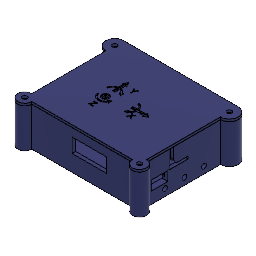
Main_Board_Box v1 (Autodesk Fusion 360 design; units mm, degrees)
part number: Utils
Autodesk Fusion 360 part; units mm, degrees
sketch "Sketch1" plane through (0, 0, 0) normal (0, 1, 0) x (1, 0, 0) in component "Bottom"
  line L0 (43.255, -32.62) -> (-43.255, -32.62) construction
  line L1 (-43.255, -32.62) -> (-43.255, 32.62) construction
  line L2 (-43.255, 32.62) -> (43.255, 32.62) construction
  line L3 (43.255, 32.62) -> (43.255, -32.62) construction
  line L4 (43.255, -32.62) -> (-43.255, 32.62) construction
  line L5 (-43.255, -32.62) -> (43.255, 32.62) construction
  line L6 (43.5, -33) -> (-43.5, -33)
  line L7 (-43.5, -33) -> (-43.5, 33)
  line L8 (-43.5, 33) -> (43.5, 33)
  line L9 (43.5, 33) -> (43.5, -33)
  line L10 (43.5, -33) -> (-43.5, 33) construction
  line L11 (-43.5, -33) -> (43.5, 33) construction
  line L12 (-43.255, -32.62) -> (-29.285, -32.62)
  line L13 (-29.285, -32.62) -> (-29.285, -28.81) construction
  circle A0 centre (-29.285, -28.81) radius 1.1
  line L14 (-29.285, -28.81) -> (29.135, -28.81) construction
  circle A1 centre (29.135, -28.81) radius 1.1
  line L15 (-29.285, -28.81) -> (-29.285, 28.34) construction
  line L16 (-43.255, 28.34) -> (-25.475, 28.34) construction
  circle A2 centre (-25.475, 28.34) radius 1.1
  line L17 (-25.475, 28.34) -> (15.165, 28.34) construction
  circle A3 centre (15.165, 28.34) radius 1.1
  line L18 (-43.255, 32.62) -> (-41.255, 32.62) construction
  line L19 (-41.255, 32.62) -> (-41.255, 40.62) construction
  line L20 (-41.255, 40.62) -> (-10.255, 40.62) construction
  line L21 (-10.255, 40.62) -> (-10.255, 32.62) construction
  line L22 (34.135, -33) -> (24.135, -33)
  line L23 (24.135, -33) -> (24.135, -27.62)
  line L24 (27.135, -24.62) -> (31.135, -24.62)
  line L25 (34.135, -27.62) -> (34.135, -33)
  arc A4 (27.135, -24.62) -> (24.135, -27.62) centre (27.135, -27.62) ccw
  arc A5 (34.135, -27.62) -> (31.135, -24.62) centre (31.135, -27.62) ccw
  line L26 (-24.285, -33) -> (-34.285, -33)
  line L27 (-34.285, -33) -> (-34.285, -27.62)
  line L28 (-31.285, -24.62) -> (-27.285, -24.62)
  line L29 (-24.285, -27.62) -> (-24.285, -33)
  arc A6 (-24.285, -27.62) -> (-27.285, -24.62) centre (-27.285, -27.62) ccw
  arc A7 (-31.285, -24.62) -> (-34.285, -27.62) centre (-31.285, -27.62) ccw
  line L30 (-15.475, 33) -> (-35.475, 33)
  line L31 (-35.475, 33) -> (-35.475, 26.68)
  line L32 (-32.475, 23.68) -> (-18.475, 23.68)
  line L33 (-15.475, 26.68) -> (-15.475, 33)
  arc A8 (-18.475, 23.68) -> (-15.475, 26.68) centre (-18.475, 26.68) ccw
  arc A9 (-35.475, 26.68) -> (-32.475, 23.68) centre (-32.475, 26.68) ccw
  line L34 (25.165, 33) -> (5.165, 33)
  line L35 (5.165, 33) -> (5.165, 26.68)
  line L36 (8.165, 23.68) -> (22.165, 23.68)
  line L37 (25.165, 26.68) -> (25.165, 33)
  arc A10 (22.165, 23.68) -> (25.165, 26.68) centre (22.165, 26.68) ccw
  arc A11 (5.165, 26.68) -> (8.165, 23.68) centre (8.165, 26.68) ccw
  line L38 (45.5, -35) -> (-45.5, -35)
  line L39 (-45.5, -35) -> (-45.5, 35)
  line L40 (45.5, 35) -> (45.5, -35)
  line L41 (45.5, -35) -> (-45.5, 35) construction
  line L42 (-45.5, -35) -> (45.5, 35) construction
  line L43 (-43.255, 35) -> (-43.255, 42.5)
  line L44 (-43.255, 42.5) -> (-8.255, 42.5)
  line L45 (-45.5, 35) -> (-43.255, 35)
  line L46 (-8.255, 35) -> (45.5, 35) construction
  line L47 (48.5, 38) -> (-48.5, -38) construction
  line L48 (-48.5, 38) -> (48.5, -38) construction
  line L49 (-5.255, 45.5) -> (-46.255, 45.5)
  circle A12 centre (48.5, 38) radius 1.4
  circle A13 centre (-48.5, 38) radius 1.4
  circle A14 centre (48.5, -38) radius 1.4
  circle A15 centre (-48.5, -38) radius 1.4
  arc A16 (42.5, -38) -> (48.5, -32) centre (48.5, -38) ccw
  line L50 (48.5, -32) -> (48.5, 30.5)
  arc A17 (-48.5, -32) -> (-42.5, -38) centre (-48.5, -38) ccw
  line L51 (-46.255, 45.5) -> (-48.5, 45.5)
  arc A18 (-48.5, 45.5) -> (-48.5, 30.5) centre (-48.5, 38) ccw
  line L52 (-42.5, -38) -> (42.5, -38)
  line L53 (-48.5, 30.5) -> (-48.5, -32)
  line L54 (-5.255, 45.5) -> (48.5, 45.5)
  line L55 (-8.255, 42.5) -> (45.5, 42.5)
  arc A19 (48.5, 30.5) -> (48.5, 45.5) centre (48.5, 38) ccw
  arc A20 (45.5, 41) -> (45.5, 35) centre (48.5, 38) ccw
  line L56 (45.5, 42.5) -> (45.5, 41)
  point P0 (29.135, -28.81)
  point P1 (-29.285, -28.81)
  point P2 (-25.475, 28.34)
  point P3 (15.165, 28.34)
  dimension "d1" = 86.51
  dimension "d2" = 65.24
  dimension "d3" = 87
  dimension "d4" = 66
  dimension "d5" = 13.97
  dimension "d6" = 3.81
  dimension "d7" = 2.2
  dimension "d8" = 58.42
  dimension "d9" = 2.2
  dimension "d10" = 57.15
  dimension "d11" = 17.78
  dimension "d12" = 2.2
  dimension "d13" = 40.64
  dimension "d14" = 2.2
  dimension "d15" = 2
  dimension "d16" = 8
  dimension "d17" = 31
  dimension "d19" = 3
  dimension "d20" = 3
  dimension "d22" = 3
  dimension "d23" = 3
  dimension "d25" = 3
  dimension "d26" = 3
  dimension "d28" = 3
  dimension "d29" = 3
  dimension "d30" = 91
  dimension "d31" = 70
  dimension "d33" = 7.5
  dimension "d34" = 97
  dimension "d35" = 76
  dimension "d39" = 2.8
  dimension "d40" = 2.8
  dimension "d41" = 2.8
  dimension "d42" = 2.8
  dimension "d43" = 6
  dimension "d44" = 6
  constraint perpendicular L0 L1
  constraint parallel L0 L2
  constraint parallel L1 L3
  constraint horizontal L0
  constraint coincident L4 origin
  constraint coincident L5 origin
  constraint perpendicular L6 L7
  constraint parallel L6 L8
  constraint parallel L7 L9
  constraint horizontal L6
  constraint coincident L10 origin
  constraint coincident L11 origin
  constraint perpendicular L1 L12
  constraint vertical L13
  constraint coincident P1 L13.end
  constraint horizontal L14
  constraint coincident P0 L14.end
  constraint vertical L15
  constraint coincident L1 L16.start
  constraint perpendicular L1 L16
  constraint coincident P2 L16.end
  constraint horizontal L17
  constraint coincident P3 L17.end
  constraint perpendicular L1 L18
  constraint perpendicular L2 L19
  constraint perpendicular L19 L20
  constraint coincident L2 L21.end
  constraint perpendicular L2 L21
  constraint perpendicular L22 L23
  constraint parallel L22 L24
  constraint parallel L23 L25
  constraint horizontal L22
  constraint coincident L6 L22.start
  constraint tangent L23 A4
  constraint tangent L24 A4
  constraint tangent L25 A5
  constraint tangent L24 A5
  constraint perpendicular L26 L27
  constraint parallel L26 L28
  constraint parallel L27 L29
  constraint horizontal L26
  constraint coincident L6 L26.start
  constraint tangent L29 A6
  constraint tangent L28 A6
  constraint tangent L27 A7
  constraint tangent L28 A7
  constraint perpendicular L30 L31
  constraint parallel L30 L32
  constraint parallel L31 L33
  constraint horizontal L30
  constraint coincident L8 L30.start
  constraint tangent L32 A8
  constraint tangent L33 A8
  constraint tangent L32 A9
  constraint tangent L31 A9
  constraint perpendicular L34 L35
  constraint parallel L34 L36
  constraint parallel L35 L37
  constraint horizontal L34
  constraint coincident L8 L34.start
  constraint tangent L36 A10
  constraint tangent L37 A10
  constraint tangent L36 A11
  constraint tangent L35 A11
  constraint perpendicular L38 L39
  constraint parallel L38 L45
  constraint parallel L39 L40
  constraint horizontal L38
  constraint coincident L41 origin
  constraint coincident L42 origin
  constraint perpendicular L20 L43
  constraint perpendicular L43 L44
  constraint collinear L45 L46
  constraint coincident L47 origin
  constraint coincident L48 origin
  constraint coincident L47.start A12.centre
  constraint coincident L48.start A13.centre
  constraint coincident L48.end A14.centre
  constraint coincident L47.end A15.centre
  constraint perpendicular L40 L54
  constraint perpendicular L40 L55
  constraint perpendicular L55 L56
  measures "d1" distance of L1.end L2.end
  measures "d2" distance of L0.end L1.end
  measures "d3" distance of L7.end L8.end
  measures "d4" distance of L6.end L7.end
  measures "d5" distance of L0.end L12.end
  measures "d6" distance of L12.end P1
  measures "d7" diameter of A0
  measures "d8" distance of P1 P0
  measures "d9" diameter of A1
  measures "d10" distance of P1 L15.end
  measures "d11" distance of L16.start P2
  measures "d12" diameter of A2
  measures "d13" distance of P2 P3
  measures "d14" diameter of A3
  measures "d15" distance of L1.end L18.end
  measures "d16" distance of L18.end L19.end
  measures "d17" distance of L19.end L20.end
  measures "d19" radius of A4
  measures "d20" radius of A5
  measures "d22" radius of A6
  measures "d23" radius of A7
  measures "d25" radius of A8
  measures "d26" radius of A9
  measures "d28" radius of A10
  measures "d29" radius of A11
  measures "d30" distance of L39.end L40.start
  measures "d31" distance of L38.end L39.end
  measures "d33" distance of L43.start L43.end
  measures "d34" distance of L47.end L48.end
  measures "d35" distance of L48.start L47.end
  measures "d39" diameter of A12
  measures "d40" diameter of A13
  measures "d41" diameter of A14
  measures "d42" diameter of A15
  measures "d43" radius of A16
  measures "d44" radius of A17
extrude "Extrude1" add sketch "Sketch1" against normal blind 2 from surface at -8 contours L6 L7 L8 L9 L23 L24 L25 A4 A5 L27 L28 L29 A6 A7 L31 L32 L33 A8 A9 L35 L36 L37 A10 A11 | L6 L22 L23 L24 L25 A4 A5 | L8 L34 L35 L36 L37 A10 A11 | L6 L26 L27 L28 L29 A6 A7 | L8 L30 L31 L32 L33 A8 A9 | L38 L39 L40 L43 L44 L45 L55 A20 L56 | L49 A16 L50 A17 L51 A18 L52 L53 L54 A19 makes body 1 in component "Bottom"
extrude "Extrude2" add sketch "Sketch1" against normal blind 8 contours L6 L22 L23 L24 L25 A4 A5 | L8 L34 L35 L36 L37 A10 A11 | L6 L26 L27 L28 L29 A6 A7 | L8 L30 L31 L32 L33 A8 A9 | L38 L39 L40 L43 L44 L45 L55 A20 L56 | L49 A16 L50 A17 L51 A18 L52 L53 L54 A19 bodies 1 in component "Bottom"
extrude "Extrude3" add sketch "Sketch1" along normal blind 2 contours L38 L39 L40 L43 L44 L45 L55 A20 L56 bodies 1 in component "Bottom"
extrude "Extrude4" add sketch "Sketch1" along normal blind 23 contours L49 A16 L50 A17 L51 A18 L52 L53 L54 A19 bodies 1 in component "Bottom"
sketch "Sketch1 (2)" plane through (0, 23, 0) normal (0, 1, 0) x (-1, 0, 0) in component "Top"
  circle A0 centre (-48.5, 38) radius 1.4 construction
  circle A1 centre (48.5, 38) radius 1.4 construction
  circle A2 centre (-48.5, -38) radius 1.4 construction
  line L0 (43.255, -42.5) -> (-45.5, -42.5)
  line L1 (-45.5, -42.5) -> (-45.5, -41)
  arc A3 (-45.5, -41) -> (-45.5, -35) centre (-48.5, -38) ccw
  line L2 (-45.5, -35) -> (-45.5, 35)
  line L3 (-45.5, 35) -> (45.5, 35)
  line L4 (45.5, 35) -> (45.5, -35)
  line L5 (45.5, -35) -> (43.255, -35)
  line L6 (43.255, -35) -> (43.255, -42.5)
  circle A4 centre (48.5, -38) radius 1.4 construction
  line L7 (-48.5, -45.5) -> (48.5, -45.5)
  arc A5 (48.5, -45.5) -> (48.5, -30.5) centre (48.5, -38) ccw
  line L8 (48.5, -30.5) -> (48.5, 32)
  arc A6 (48.5, 32) -> (42.5, 38) centre (48.5, 38) ccw
  line L9 (42.5, 38) -> (-42.5, 38)
  arc A7 (-42.5, 38) -> (-48.5, 32) centre (-48.5, 38) ccw
  line L10 (-48.5, 32) -> (-48.5, -30.5)
  arc A8 (-48.5, -30.5) -> (-48.5, -45.5) centre (-48.5, -38) ccw
  line L11 (45.5, 35) -> (45, 35)
  line L12 (45.5, 34.5) -> (45.5, 35)
  line L13 (-45.5, 35) -> (-45, 35)
  line L14 (-45.5, 34.5) -> (-45.5, 35)
  line L15 (45.5, -35) -> (45, -35)
  line L16 (45.5, -34.5) -> (45.5, -35)
  line L17 (42.755, -35) -> (42.755, -34.5)
  line L18 (42.755, -34.5) -> (43.255, -34.5)
  line L19 (43.255, -42.5) -> (42.755, -42.5)
  line L20 (43.255, -42) -> (43.255, -42.5)
  line L21 (-45.5, -34.5) -> (-45.5, -35)
  line L22 (-45, -41.5) -> (-45, -42)
  line L23 (-45, -42.5) -> (-45.5, -42.5)
  line L24 (-45.5, -42.5) -> (-45.5, -41)
  arc A9 (-45, -41.5) -> (-45, -34.5) centre (-48.5, -38) ccw
  line L25 (-45, -42) -> (42.755, -42)
  line L26 (42.755, -42) -> (42.755, -35)
  line L27 (43.255, -34.5) -> (45, -34.5)
  line L28 (45, -34.5) -> (45, 34.5)
  line L29 (45, 34.5) -> (-45, 34.5)
  line L30 (-45, 34.5) -> (-45, -34.5)
  line L31 (-47, -42.5) -> (-47, -40)
  line L32 (40.755, -40) -> (40.755, -35)
  line L33 (40.755, -35) -> (40.755, -32.5)
  line L34 (40.755, -32.5) -> (43, -32.5)
  line L35 (43, -32.5) -> (43, 32.5)
  line L36 (43, 32.5) -> (-43, 32.5)
  line L37 (-43, 32.5) -> (-43, -33.7516)
  arc A10 (-41.8443, -40) -> (-43, -33.7516) centre (-48.5, -38) ccw
  line L38 (-47, -40) -> (-44.7583, -40)
  line L39 (-41.8443, -40) -> (40.755, -40)
  circle A11 centre (48.5, -38) radius 2
  circle A12 centre (48.5, 38) radius 2
  circle A13 centre (-48.5, 38) radius 2
  circle A14 centre (-48.5, -38) radius 2
  dimension "d56" = 0.5
  dimension "d57" = 0.5
  dimension "d58" = 0.5
  dimension "d59" = 0.5
  dimension "d60" = 0.5
  dimension "d61" = 0.5
  dimension "d62" = 0.5
  dimension "d63" = 0.5
  dimension "d64" = 0.5
  dimension "d65" = 0.5
  dimension "d67" = 0.5
  dimension "d70" = 0.5
  dimension "d76" = 4
  dimension "d77" = 4
  dimension "d78" = 4
  dimension "d79" = 4
  constraint horizontal L11
  constraint vertical L12
  constraint coincident L3.end L4.start
  constraint horizontal L13
  constraint vertical L14
  constraint coincident L2.end L3.start
  constraint horizontal L15
  constraint vertical L16
  constraint coincident L4.end L5.start
  constraint vertical L17
  constraint horizontal L18
  constraint horizontal L19
  constraint vertical L20
  constraint coincident L0.start L6.end
  constraint vertical L21
  constraint coincident A3.end L2.start
  constraint vertical L22
  constraint horizontal L23
  constraint vertical L24
  constraint coincident L1.end A3.start
  constraint coincident L0 L23.start
  constraint coincident A2.centre A3.centre
  constraint parallel L25 L38
  constraint parallel L26 L32
  constraint parallel L17 L33
  constraint parallel L18 L34
  constraint parallel L28 L35
  constraint parallel L29 L36
  constraint parallel L30 L37
  constraint coincident A10.start L38
  constraint collinear L38 L39
  constraint coincident A3 L38.end
  constraint concentric A4 A11
  constraint concentric A1 A12
  constraint concentric A0 A13
  constraint concentric A9 A14
  measures "d56" distance of L3.end L12.start
  measures "d57" distance of L3.end L11.end
  measures "d58" distance of L2.end L14.start
  measures "d59" distance of L2.end L13.end
  measures "d60" distance of L4.end L15.end
  measures "d61" distance of L4.end L16.start
  measures "d62" distance of L5.end L17.start
  measures "d63" distance of L5.end L18.end
  measures "d64" distance of L0.start L19.end
  measures "d65" distance of L0.start L20.start
  measures "d67" distance of A3.end L21.start
  measures "d70" distance of L23.start L22.end
  measures "d76" diameter of A11
  measures "d77" diameter of A12
  measures "d78" diameter of A13
  measures "d79" diameter of A14
extrude "Extrude1'" add sketch "Sketch1 (2)" against normal blind 3 separate body contours L17 L18 L22 A9 L25 L26 L27 L28 L29 L30 makes body 2 in component "Top"
extrude "Extrude2'" add sketch "Sketch1 (2)" along normal blind 2 contours L0 L1 A3 L2 L3 L4 L5 L6 L11 L12 L13 L14 L15 L16 L19 L20 L21 L23 L24 | L7 A5 L8 A6 L9 A7 L10 A8 | L17 L18 L22 A9 L25 L26 L27 L28 L29 L30 | L32 L33 L34 L35 L36 L37 A10 L39 bodies 2 in component "Top"
sketch "Sketch2" plane through (48.5, 0, 0) normal (1, 0, 0) x (0, 0, -1) in component "Bottom"
  line L0 (-32, 23) -> (-32, -10)
  line L1 (-32, -10) -> (30.5, -10)
  line L2 (30.5, -10) -> (30.5, 23)
  line L3 (30.5, 23) -> (-32, 23)
  line L4 (-32, 0) -> (30.5, 0)
  line L5 (33, 2) -> (-33, 2) construction
  line L6 (35, 0) -> (-35, 0)
  line L7 (-33, -8) -> (-33, 2)
  line L8 (-33, 0) -> (-28, 0)
  line L9 (-33, 0) -> (-14, 0)
  line L10 (-28, 0) -> (-14, 0)
  line L11 (-14, 0) -> (-14, 8)
  line L12 (-14, 8) -> (-28, 8)
  line L13 (-28, 8) -> (-28, 0)
  line L14 (-13, 8) -> (3, 8)
  line L15 (3, 8) -> (3, 10)
  line L16 (3, 10) -> (-5.4645, 10)
  line L17 (-13, 10) -> (-13, 8)
  line L18 (-13, 8) -> (-9, 8)
  line L19 (-9, 23) -> (-13, 23)
  line L20 (-13, 23) -> (-13, 8)
  arc A0 (-9, 13.5355) -> (-5.4645, 10) centre (-5.4645, 13.5355) ccw
  line L21 (-9, 13.5355) -> (-9, 23)
  line L22 (33, 2) -> (33, -8)
  line L23 (33, -8) -> (-33, -8)
  line L24 (-33, -8) -> (-33, 2)
  line L25 (-33, 2) -> (33, 2)
  line L26 (-33, 0) -> (33, -8) construction
  line L27 (33, 0) -> (-33, -8) construction
  line L28 (0, 0) -> (-33, -8) construction
  line L29 (-33, 0) -> (0, -8) construction
  line L30 (33, 0) -> (0, -8) construction
  line L31 (0, 0) -> (33, -8) construction
  circle A1 centre (-16.5, -4) radius 2
  circle A2 centre (0, -4) radius 2
  circle A3 centre (16.5, -4) radius 2
  dimension "d82" = 5
  dimension "d83" = 19
  dimension "d84" = 8
  dimension "d88" = 1
  dimension "d89" = 16
  dimension "d90" = 2
  dimension "d91" = 4
  dimension "d92" = 4
  dimension "d93" = 4
  dimension "d94" = 4
  dimension "d69_1" = 0
  dimension "d73_1" = 0
  dimension "d129_1" = 0
  constraint coincident L6 L8.start
  constraint coincident L7 L8.start
  constraint perpendicular L7 L8
  constraint parallel L6 L9
  constraint horizontal L10
  constraint vertical L11
  constraint horizontal L12
  constraint vertical L13
  constraint horizontal L14
  constraint vertical L15
  constraint horizontal L16
  constraint vertical L17
  constraint horizontal L18
  constraint horizontal L19
  constraint vertical L20
  constraint coincident L3 L19.start
  constraint tangent L16 A0
  constraint coincident L22.end L23.start
  constraint coincident L6 L27.start
  constraint coincident L22 L27.start
  constraint coincident L7.start L23.end
  constraint coincident L28.start L31.start
  constraint midpoint L23 L29.end
  constraint midpoint L28 A1.centre
  constraint midpoint L26 A2.centre
  constraint midpoint L30 A3.centre
  measures "d82" distance of L8.start L8.end
  measures "d83" distance of L8.start L9.end
  measures "d84" distance of L8.end L12.end
  measures "d88" distance of L11.end L14.start
  measures "d89" distance of L14.start L14.end
  measures "d90" distance of L14.start L17.start
  measures "d91" distance of L14.start L18.end
  measures "d92" diameter of A1
  measures "d93" diameter of A2
  measures "d94" diameter of A3
extrude "Extrude5" cut sketch "Sketch2" against normal blind 10 contours L4 L6 L9 L10 L11 L13 L25 | L11 L12 L13 L25 bodies 1 in component "Bottom"
extrude "Extrude6" cut sketch "Sketch2" against normal blind 5 contours L3 L14 L15 L16 L17 L18 L19 L20 A0 L21 bodies 1 in component "Bottom"
extrude "Extrude7" cut sketch "Sketch2" against normal blind 107 contours A1 | A2 | A3 bodies 1 in component "Bottom"
sketch "Sketch3" plane through (0, 0, 38) normal (0, 0, 1) x (1, 0, 0) in component "Bottom"
  line L0 (-42.5, 23) -> (-42.5, -10)
  line L1 (-42.5, -10) -> (42.5, -10)
  line L2 (42.5, -10) -> (42.5, 23)
  line L3 (42.5, 23) -> (-42.5, 23)
  line L4 (-42.5, 0) -> (42.5, 0)
  line L5 (43.5, 0) -> (20.5, 0)
  line L6 (20.5, 0) -> (20.5, 4)
  line L7 (43.5, 0) -> (-8.5, 0)
  line L8 (20.5, 4) -> (-8.5, 4)
  line L9 (-8.5, 4) -> (-8.5, 16)
  line L10 (-8.5, 16) -> (20.5, 16)
  line L11 (20.5, 16) -> (20.5, 4)
  point P0 (43.5, 0)
  dimension "d99" = 23
  dimension "d100" = 4
  dimension "d101" = 52
  dimension "d102" = 12
  constraint coincident P0 L5.start
  constraint perpendicular L2 L5
  constraint perpendicular L4 L6
  constraint perpendicular L6 L7
  constraint horizontal L8
  constraint vertical L9
  constraint horizontal L10
  constraint vertical L11
  measures "d99" distance of P0 L5.end
  measures "d100" distance of L5.end L6.end
  measures "d101" distance of P0 L7.end
  measures "d102" distance of L6.end L10.end
extrude "Extrude8" cut sketch "Sketch3" against normal blind 7 contours L8 L9 L10 L11 bodies 1 in component "Bottom"
sketch "Sketch6" plane through (0, 25, 0) normal (0, 1, 0) x (-1, 0, 0) in component "Utils"
  line L0 (15.1244, 3.1244) -> (21.0332, 4.1662) construction
  line L1 (15.1244, 3.1244) -> (15.1244, 8.1244) construction
  line L2 (15.1244, 3.1244) -> (10.7942, 5.6244) construction
  line L3 (15.1244, 3.1244) -> (15.1244, 8.1244) construction
  line L4 (15.1244, 3.1244) -> (15.1244, 9.1244) construction
  line L5 (9.0622, 6.6244) -> (9.0622, 3.6244)
  line L6 (15.1244, 3.1244) -> (20.0484, 3.9926) construction
  line L7 (11.6603, 5.1244) -> (9.0622, 3.6244)
  line L8 (15.1244, 6.1244) -> (15.1244, 8.1244)
  arc A0 (15.1244, 8.1244) -> (10.7942, 5.6244) centre (15.1244, 3.1244) ccw
  line L9 (15.1244, 3.1244) -> (15.1244, 6.1244) construction
  line L10 (15.1244, 8.1244) -> (15.1244, 9.1244) construction
  line L11 (20.0484, 3.9926) -> (21.0332, 4.1662)
  line L12 (9.9282, 6.1244) -> (9.0622, 6.6244)
  circle A1 centre (15.1244, 3.1244) radius 1
  arc A2 (21.0332, 4.1662) -> (15.1244, 9.1244) centre (15.1244, 3.1244) ccw
  line L13 (10.7942, 5.6244) -> (11.6603, 5.1244)
  circle A3 centre (15.1244, 3.1244) radius 3
  arc A4 (15.1244, 9.1244) -> (9.9282, 6.1244) centre (15.1244, 3.1244) ccw
  arc A5 (20.0484, 3.9926) -> (15.1244, 8.1244) centre (15.1244, 3.1244) ccw
  line L14 (15.1244, 3.1244) -> (15.1244, 9.1244) construction
  line L15 (15.1244, 3.1244) -> (9.9282, 6.1244) construction
  circle A6 centre (15.1244, 3.1244) radius 2
  line L16 (16.9519, 15.6272) -> (13.5564, 15.6272) construction
  line L17 (13.5564, 15.6272) -> (13.5564, 9.6272) construction
  line L18 (13.5564, 9.6272) -> (16.9519, 9.6272) construction
  line L19 (16.9519, 9.6272) -> (16.9519, 15.6272) construction
  line L20 (0, 0) -> (-4, 0) construction
  line L21 (-4, 0) -> (-4, -1)
  line L22 (-4, 0) -> (-4, 1)
  line L23 (-4, -1) -> (-15, -1)
  line L24 (-15, -1) -> (-15, -2)
  line L25 (-4, 1) -> (-15, 1)
  line L26 (-15, 1) -> (-15, 2)
  line L27 (-15, -2) -> (-18.4641, 0)
  line L28 (-15, 2) -> (-18.4641, 0)
  line L29 (-8.0481, 8.6272) -> (-11.9856, 8.6272) construction
  line L30 (-11.9856, 8.6272) -> (-11.9856, 2.6272) construction
  line L31 (-11.9856, 2.6272) -> (-8.0481, 2.6272) construction
  line L32 (-8.0481, 2.6272) -> (-8.0481, 8.6272) construction
  arc A7 (-5.5622, 4.2679) -> (-7.6024, 2.0322) centre (-3.0622, -0.0622) ccw
  line L33 (-6.5622, 6) -> (-3.5622, 6)
  line L34 (-3.9304, -4.9862) -> (-4.1041, -5.971)
  arc A8 (-6.0622, 5.134) -> (-8.5104, 2.4511) centre (-3.0622, -0.0622) ccw
  line L35 (-6.0622, 5.134) -> (-6.5622, 6)
  line L36 (-5.0622, 3.4019) -> (-3.5622, 6)
  line L37 (-5.5622, 4.2679) -> (-5.0622, 3.4019)
  line L38 (16.3923, -4.1436) -> (16.3923, -13.1436)
  line L39 (17.3923, -13.1436) -> (15.3923, -16.6077)
  line L40 (16.3923, -13.1436) -> (17.3923, -13.1436)
  line L41 (14.3923, -4.1436) -> (14.3923, -13.1436)
  line L42 (14.3923, -13.1436) -> (13.3923, -13.1436)
  arc A9 (10.2583, -6.2058) -> (12.9412, -8.654) centre (15.4545, -3.2058) ccw
  line L43 (20.3785, -4.074) -> (21.3633, -4.2477)
  line L44 (15.3923, -4.1436) -> (14.3923, -4.1436)
  line L45 (11.9904, -5.2058) -> (9.3923, -3.7058)
  arc A10 (11.1244, -5.7058) -> (13.3601, -7.746) centre (15.4545, -3.2058) ccw
  line L46 (13.3923, -13.1436) -> (15.3923, -16.6077)
  line L47 (15.3923, -4.1436) -> (16.3923, -4.1436)
  line L48 (11.1244, -5.7058) -> (11.9904, -5.2058)
  line L49 (9.3923, -6.7058) -> (9.3923, -3.7058)
  line L50 (10.2583, -6.2058) -> (9.3923, -6.7058)
  line L51 (8.9519, -10.3728) -> (5.0144, -10.3728) construction
  line L52 (5.0144, -10.3728) -> (5.0144, -16.3728) construction
  line L53 (5.0144, -16.3728) -> (8.9519, -16.3728) construction
  line L54 (8.9519, -16.3728) -> (8.9519, -10.3728) construction
  arc A11 (-7.6024, 2.0322) -> (-7.9481, 1) centre (-3.0622, -0.0622) ccw
  arc A12 (-7.9734, -1) -> (-3.9304, -4.9862) centre (-3.0622, -0.0622) ccw
  arc A13 (-7.9481, 1) -> (-7.9734, -1) centre (-3.0622, -0.0622) ccw construction
  arc A14 (-8.5104, 2.4511) -> (-8.9674, 1) centre (-3.0622, -0.0622) ccw
  arc A15 (-8.9884, -1) -> (-4.1041, -5.971) centre (-3.0622, -0.0622) ccw
  arc A16 (-8.9674, 1) -> (-8.9884, -1) centre (-3.0622, -0.0622) ccw construction
  arc A17 (12.9412, -8.654) -> (14.3923, -9.111) centre (15.4545, -3.2058) ccw
  arc A18 (16.3923, -9.132) -> (21.3633, -4.2477) centre (15.4545, -3.2058) ccw
  arc A19 (14.3923, -9.111) -> (16.3923, -9.132) centre (15.4545, -3.2058) ccw construction
  arc A20 (13.3601, -7.746) -> (14.3923, -8.0916) centre (15.4545, -3.2058) ccw
  arc A21 (16.3923, -8.117) -> (20.3785, -4.074) centre (15.4545, -3.2058) ccw
  arc A22 (14.3923, -8.0916) -> (16.3923, -8.117) centre (15.4545, -3.2058) ccw construction
  circle A23 centre (-48.5, -38) radius 2
  circle A24 centre (-48.5, 38) radius 2
  circle A25 centre (48.5, -38) radius 2
  circle A26 centre (48.5, 38) radius 2
  arc A27 (-48.5, -30.5) -> (-48.5, -45.5) centre (-48.5, -38) ccw
  line L55 (-48.5, -45.5) -> (48.5, -45.5)
  arc A28 (48.5, -45.5) -> (48.5, -30.5) centre (48.5, -38) ccw
  line L56 (48.5, -30.5) -> (48.5, 32)
  arc A29 (48.5, 32) -> (42.5, 38) centre (48.5, 38) ccw
  line L57 (42.5, 38) -> (-42.5, 38)
  arc A30 (-42.5, 38) -> (-48.5, 32) centre (-48.5, 38) ccw
  line L58 (-48.5, 32) -> (-48.5, -30.5)
  circle A31 centre (-48.5, -38) radius 2
  circle A32 centre (-48.5, 38) radius 2
  circle A33 centre (48.5, -38) radius 2
  circle A34 centre (48.5, 38) radius 2
  arc A35 (-48.5, -30.5) -> (-48.5, -45.5) centre (-48.5, -38) ccw
  line L59 (-48.5, -45.5) -> (48.5, -45.5)
  arc A36 (48.5, -45.5) -> (48.5, -30.5) centre (48.5, -38) ccw
  line L60 (48.5, -30.5) -> (48.5, 32)
  arc A37 (48.5, 32) -> (42.5, 38) centre (48.5, 38) ccw
  line L61 (42.5, 38) -> (-42.5, 38)
  arc A38 (-42.5, 38) -> (-48.5, 32) centre (-48.5, 38) ccw
  line L62 (-48.5, 32) -> (-48.5, -30.5)
  circle A39 centre (-48.5, -38) radius 2
  circle A40 centre (-48.5, 38) radius 2
  circle A41 centre (48.5, -38) radius 2
  circle A42 centre (48.5, 38) radius 2
  arc A43 (-48.5, -30.5) -> (-48.5, -45.5) centre (-48.5, -38) ccw
  line L63 (-48.5, -45.5) -> (48.5, -45.5)
  arc A44 (48.5, -45.5) -> (48.5, -30.5) centre (48.5, -38) ccw
  line L64 (48.5, -30.5) -> (48.5, 32)
  arc A45 (48.5, 32) -> (42.5, 38) centre (48.5, 38) ccw
  line L65 (42.5, 38) -> (-42.5, 38)
  arc A46 (-42.5, 38) -> (-48.5, 32) centre (-48.5, 38) ccw
  line L66 (-48.5, 32) -> (-48.5, -30.5)
  dimension "d101_1" = 2
  dimension "d102_1" = 4
  dimension "d103_1" = 6
  dimension "d104_1" = 2
  dimension "d105_1" = 80
  dimension "d106_1" = 60
  dimension "d107_1" = 1
  dimension "d108_1" = 80
  dimension "d109_1" = 60
  dimension "d110_1" = 1
  dimension "d111_1" = 1
  dimension "d112_1" = 4
  dimension "d113_1" = 1
  dimension "d114_1" = 1
  dimension "d115_1" = 11
  dimension "d116_1" = 1
  dimension "d117_1" = 11
  dimension "d118_1" = 1
  dimension "d122_1" = 1
  dimension "d123_1" = 1
  dimension "d125_1" = 1
  dimension "d127_1" = 1
  text T0 "Z" font "Arial" height 6 align ink ink in box 0 x 0 at (16.9519, 15.6272) x (-1, 0) y (0, -1) spacing 1 height is em
  text T1 "X" font "Arial" height 6 align ink ink in box 0 x 0 at (-8.0481, 8.6272) x (-1, 0) y (0, -1) spacing 1 height is em
  text T2 "Y" font "Arial" height 6 align ink ink in box 0 x 0 at (8.9519, -10.3728) x (-1, 0) y (0, -1) spacing 1 height is em
  constraint concentric A1 A6
  constraint concentric A1 A3
  constraint coincident L0.start L1.start
  constraint coincident L8.start A3
  constraint parallel L8 L9
  constraint parallel L1 L10
  constraint parallel L2 L13
  constraint parallel L12 L15
  constraint perpendicular L16 L17
  constraint parallel L16 L18
  constraint parallel L17 L19
  constraint coincident L20.start origin
  constraint perpendicular L20 L21
  constraint perpendicular L20 L22
  constraint perpendicular L21 L23
  constraint perpendicular L23 L24
  constraint perpendicular L22 L25
  constraint perpendicular L25 L26
  constraint perpendicular L29 L30
  constraint parallel L29 L31
  constraint parallel L30 L32
  constraint perpendicular L38 L47
  constraint perpendicular L38 L40
  constraint perpendicular L41 L44
  constraint perpendicular L51 L52
  constraint parallel L51 L53
  constraint parallel L52 L54
  constraint coincident L25 A11.end
  constraint coincident L23 A12.start
  constraint concentric A11 A12
  constraint concentric A11 A13
  constraint coincident L25 A14.end
  constraint coincident L23 A15.start
  constraint concentric A14 A15
  constraint concentric A14 A16
  constraint coincident L41 A17.end
  constraint coincident L38 A18.start
  constraint concentric A17 A18
  constraint concentric A17 A19
  constraint coincident L41 A20.end
  constraint coincident L38 A21.start
  constraint concentric A20 A21
  constraint concentric A20 A22
  measures "d101_1" diameter of A1
  measures "d102_1" diameter of A6
  measures "d103_1" diameter of A3
  measures "d104_1" distance of L8.start L1.end
  measures "d105_1" angle of L1 L6
  measures "d106_1" angle of L2 L3
  measures "d107_1" distance of L4.end L1.end
  measures "d108_1" angle of L0 L4
  measures "d109_1" angle of L14 L15
  measures "d110_1" distance of L2.end L7.start
  measures "d111_1" distance of L12.start L5.start
  measures "d112_1" distance of L20.start L20.end
  measures "d113_1" distance of L20.end L21.end
  measures "d114_1" distance of L20.end L22.end
  measures "d115_1" distance of L21.end L23.end
  measures "d116_1" distance of L23.end L24.end
  measures "d117_1" distance of L22.end L25.end
  measures "d118_1" distance of L25.end L26.end
  measures "d122_1" distance of L44.start L38.start
  measures "d123_1" distance of L41.start L44.start
  measures "d125_1" distance of L39.start L38.end
  measures "d127_1" distance of L42.end L41.end
extrude "Extrude3'" cut sketch "Sketch6" sketch "Sketch6" against normal blind 1 contours L5 L7 A0 L11 L12 A2 L13 A4 A5 | A1 | A3 | L21 L22 L23 L24 L25 L26 L27 L28 | L23 L34 A12 A15 | L25 A7 L33 A8 L35 L36 L37 A11 A14 | L38 L39 L40 L41 L42 L44 L46 L47 | L38 L43 A18 A21 | L41 A9 L45 A10 L48 L49 L50 A17 A20 of sketch 2 text T0 T2 T1 bodies 2 in component "Top"
extrude "Extrude9" add sketch "Sketch1" against normal blind 2 from surface at -8 contours A0 | A1 | A2 | A3 bodies 1 in component "Bottom"
extrude "Extrude10" add sketch "Sketch1" against normal blind 2 from surface at -8 contours A12 | A13 | A14 | A15 bodies 1 in component "Bottom"
component "Bottom" placed x (1, 0, 0) y (0, 1, 0) z (0, 0, 1) at (0, 0, 0)
component "Top" placed x (1, 0, 0) y (0, 1, 0) z (0, 0, 1) at (0, 0, 0)
component "Utils" placed x (1, 0, 0) y (0, 1, 0) z (0, 0, 1) at (0, 0, 0)
equation "d102 = 15 mm - 3 mm"
equation "d66_1 = -4.00 mm"
equation "d68_1 = 3.00 mm"
equation "d71_1 = 0.0 deg"
equation "d72_1 = 1.00 mm"
equation "d128_1 = -1 mm"
